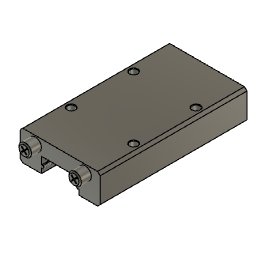
_WozekMGN15H.34389aef-dfec-4a68-be90-59f823977ef3 (Autodesk Fusion 360 design; units mm, degrees)
Autodesk Fusion 360 part; units mm, degrees
sketch "Sketch1" plane through (0, 0, 0) normal (0, 1, 0) x (1, 0, 0)
  line L0 (0, 0) -> (16, 0)
  line L1 (16, 0) -> (16, 12)
  line L2 (16, 12) -> (7.5, 12)
  line L3 (7.5, 6) -> (0, 6)
  line L4 (7.5, 12) -> (7.5, 10)
  line L5 (7.5, 10) -> (7, 10)
  line L6 (6.5, 9.5) -> (6.5, 9.5)
  line L7 (7, 9) -> (7.5, 9)
  line L8 (7.5, 9) -> (7.5, 6)
  arc A0 (6.5, 9.5) -> (7, 9) centre (7, 9.5) ccw
  arc A1 (7, 10) -> (6.5, 9.5) centre (7, 9.5) ccw
  line L9 (-7, 9) -> (-7.5, 9)
  line L10 (-7.5, 10) -> (-7, 10)
  arc A2 (-6.5, 9.5) -> (-7, 10) centre (-7, 9.5) ccw
  arc A3 (-7, 9) -> (-6.5, 9.5) centre (-7, 9.5) ccw
  line L11 (-16, 12) -> (-7.5, 12)
  line L12 (-16, 0) -> (-16, 12)
  line L13 (-6.5, 9.5) -> (-6.5, 9.5)
  line L14 (0, 0) -> (-16, 0)
  line L15 (-7.5, 6) -> (0, 6)
  line L16 (-7.5, 12) -> (-7.5, 10)
  line L17 (-7.5, 9) -> (-7.5, 6)
  point P0 (6.5, 10)
  point P1 (6.5, 9)
  point P2 (-6.5, 9)
  point P3 (-6.5, 10)
  dimension "d1" = 16
  dimension "d2" = 12
  dimension "d3" = 8.5
  dimension "d4" = 6
  dimension "d5" = 7.5
  dimension "d6" = 1
  dimension "d7" = 1
  dimension "d8" = 1
  dimension "d9" = 0.5
  dimension "d10" = 0.5
  constraint coincident L0.start L14.start
  constraint horizontal L0
  constraint perpendicular L0 L1
  constraint perpendicular L1 L2
  constraint perpendicular L2 L4
  constraint perpendicular L4 L5
  constraint perpendicular L3 L8
  constraint coincident P1 L7
  constraint tangent L7 A0
  constraint coincident P0 L5
  constraint coincident P0 L6
  constraint tangent L5 A1
  measures "d1" distance of L0.start L0.end
  measures "d2" distance of L0.end L1.end
  measures "d3" distance of L1.end L2.end
  measures "d4" distance of L2.end L3.start
  measures "d5" distance of L3.start L3.end
  measures "d6" distance of L4.end P0
  measures "d7" distance of P0 P1
  measures "d8" distance of P1 L7.end
  measures "d9" radius of A0
  measures "d10" radius of A1
extrude "Extrude1" add sketch "Sketch1" along normal blind 58.8
sketch "Sketch2" plane through (0, 0, 0) normal (0, 0, 1) x (-1, 0, 0)
  line L0 (16, 0) -> (-16, 0)
  line L1 (-16, 0) -> (-16, -58.8)
  line L2 (-16, -58.8) -> (16, -58.8)
  line L3 (16, -58.8) -> (16, 0)
  line L4 (0, -29.4) -> (-12.5, -29.4)
  line L5 (-12.5, -29.4) -> (-12.5, -41.9)
  line L6 (-12.5, -41.9) -> (0, -41.9)
  line L7 (0, -41.9) -> (0, -29.4)
  circle A0 centre (-12.5, -41.9) radius 1.5
  circle A1 centre (12.5, -41.9) radius 1.5
  circle A2 centre (12.5, -16.9) radius 1.5
  circle A3 centre (-12.5, -16.9) radius 1.5
  dimension "d13" = 12.5
  dimension "d14" = 12.5
  dimension "d15" = 3
  constraint horizontal L4
  constraint vertical L5
  constraint horizontal L6
  constraint vertical L7
  constraint coincident L5.end L6.start
  constraint symmetric L7 A0 A1
  constraint symmetric L4 A0 A3
  constraint symmetric L4 A1 A2
  measures "d13" distance of L4.start L4.end
  measures "d14" distance of L4.start L6.end
  measures "d15" diameter of A0
extrude "Extrude2" cut sketch "Sketch2" against normal blind 6 contours L5 L6 A0 | L5 L6 A0 | A1 | A2 | A3
chamfer "Chamfer1" distance 1 angle 45 4 edges at (-16, 29.4, 0) (-16, 29.4, -12) (16, 29.4, 0) (16, 29.4, -12)
chamfer "Chamfer2" distance 0.2 angle 45 4 edges at (-11.1015, 41.3576, 0) (13.8985, 41.3576, 0) (13.8985, 16.3576, 0) (-11.1015, 16.3576, 0)
sketch "Sketch3" plane through (0, 0, 0) normal (0, -1, 0) x (1, 0, 0)
  line L0 (15, -12) -> (16, -11)
  line L1 (16, -11) -> (16, -1)
  line L2 (16, -1) -> (15, 0)
  line L3 (15, 0) -> (-15, 0)
  line L4 (-15, 0) -> (-16, -1)
  line L5 (-16, -1) -> (-16, -11)
  line L6 (-16, -11) -> (-15, -12)
  line L7 (-15, -12) -> (-7.5, -12)
  line L8 (-7.5, -12) -> (-7.5, -10)
  line L9 (-7.5, -10) -> (-7, -10)
  arc A0 (-7, -10) -> (-7, -9) centre (-7, -9.5) ccw
  line L10 (-7, -9) -> (-7.5, -9)
  line L11 (-7.5, -9) -> (-7.5, -6)
  line L12 (-7.5, -6) -> (7.5, -6)
  line L13 (7.5, -6) -> (7.5, -9)
  line L14 (7.5, -9) -> (7, -9)
  arc A1 (7, -9) -> (7, -10) centre (7, -9.5) ccw
  line L15 (7, -10) -> (7.5, -10)
  line L16 (7.5, -10) -> (7.5, -12)
  line L17 (7.5, -12) -> (15, -12)
  circle A2 centre (-10, -3.0186) radius 2.5
  circle A3 centre (10, -3.0186) radius 2.5
  dimension "d22" = 5
  measures "d22" diameter of A2
extrude "Extrude3" add sketch "Sketch3" along normal blind 4.5 contours A2 | A3
chamfer "Chamfer3" distance 0.5 angle 45 2 edges at (-12.3308, -4.5, -3.9226) (7.6692, -4.5, -3.9226)
sketch "Sketch4" plane through (0, -4.5, 0) normal (0, -1, 0) x (1, 0, 0)
  circle A0 centre (-10, -3.0186) radius 2
  line L0 (-11.0354, -2.0354) -> (-10.9646, -1.9646)
  line L1 (-9.0012, -1.9676) -> (-8.9312, -2.039)
  line L2 (-11.035, -3.9643) -> (-10.965, -4.0357)
  line L3 (-9.0354, -4.0354) -> (-8.9646, -3.9646)
  line L4 (-11.0337, -3.8229) -> (-10.2039, -3.0082)
  line L5 (-9.9898, -2.7981) -> (-9.1426, -1.9663)
  line L6 (-10.8232, -1.9646) -> (-9.9898, -2.7981)
  line L7 (-9.7777, -3.0102) -> (-8.9646, -3.8232)
  line L8 (-10.8236, -4.037) -> (-9.9918, -3.2204)
  line L9 (-9.7777, -3.0102) -> (-8.9325, -2.1804)
  line L10 (-11.0354, -2.1768) -> (-10.2039, -3.0082)
  line L11 (-9.9918, -3.2204) -> (-9.1768, -4.0354)
  arc A1 (-11.0354, -2.0354) -> (-11.0354, -2.1768) centre (-10.9646, -2.1061) ccw
  arc A2 (-10.8232, -1.9646) -> (-10.9646, -1.9646) centre (-10.8939, -2.0354) ccw
  arc A3 (-9.0012, -1.9676) -> (-9.1426, -1.9663) centre (-9.0726, -2.0377) ccw
  arc A4 (-8.9325, -2.1804) -> (-8.9312, -2.039) centre (-9.0025, -2.109) ccw
  arc A5 (-8.9646, -3.9646) -> (-8.9646, -3.8232) centre (-9.0354, -3.8939) ccw
  arc A6 (-9.1768, -4.0354) -> (-9.0354, -4.0354) centre (-9.1061, -3.9646) ccw
  arc A7 (-10.965, -4.0357) -> (-10.8236, -4.037) centre (-10.8936, -3.9656) ccw
  arc A8 (-11.0337, -3.8229) -> (-11.035, -3.9643) centre (-10.9637, -3.8943) ccw
  arc A9 (11.0354, -2.1768) -> (11.0354, -2.0354) centre (10.9646, -2.1061) ccw
  line L12 (11.035, -3.9643) -> (10.965, -4.0357)
  line L13 (9.7777, -3.0102) -> (8.9325, -2.1804)
  line L14 (11.0354, -2.0354) -> (10.9646, -1.9646)
  line L15 (9.9898, -2.7981) -> (9.1426, -1.9663)
  arc A10 (8.9646, -3.8232) -> (8.9646, -3.9646) centre (9.0354, -3.8939) ccw
  arc A11 (8.9312, -2.039) -> (8.9325, -2.1804) centre (9.0025, -2.109) ccw
  line L16 (9.9918, -3.2204) -> (9.1768, -4.0354)
  arc A12 (10.8236, -4.037) -> (10.965, -4.0357) centre (10.8936, -3.9656) ccw
  arc A13 (9.0354, -4.0354) -> (9.1768, -4.0354) centre (9.1061, -3.9646) ccw
  arc A14 (11.035, -3.9643) -> (11.0337, -3.8229) centre (10.9637, -3.8943) ccw
  line L17 (10.8236, -4.037) -> (9.9918, -3.2204)
  arc A15 (9.1426, -1.9663) -> (9.0012, -1.9676) centre (9.0726, -2.0377) ccw
  line L18 (10.8232, -1.9646) -> (9.9898, -2.7981)
  arc A16 (10.9646, -1.9646) -> (10.8232, -1.9646) centre (10.8939, -2.0354) ccw
  line L19 (11.0354, -2.1768) -> (10.2039, -3.0082)
  line L20 (9.0012, -1.9676) -> (8.9312, -2.039)
  line L21 (11.0337, -3.8229) -> (10.2039, -3.0082)
  line L22 (9.7777, -3.0102) -> (8.9646, -3.8232)
  line L23 (9.0354, -4.0354) -> (8.9646, -3.9646)
  point P0 (10, -3.0186)
  dimension "d30" = 0.1
  dimension "d31" = 0.1
  constraint perpendicular L0 L6
  constraint perpendicular L1 L8
  constraint perpendicular L2 L8
  constraint perpendicular L3 L6
  constraint collinear L4 L5
  constraint coincident L7.start L8
  constraint collinear L6 L7
  constraint coincident L8.end L10
  constraint collinear L8 L9
  constraint collinear L10 L11
  constraint tangent L0 A1
  constraint tangent L10 A1
  constraint tangent L0 A2
  constraint tangent L6 A2
  constraint tangent L1 A3
  constraint tangent L5 A3
  constraint equal A2 A3
  constraint tangent L1 A4
  constraint tangent L9 A4
  constraint equal A2 A4
  constraint tangent L3 A5
  constraint tangent L7 A5
  constraint equal A2 A5
  constraint tangent L3 A6
  constraint tangent L11 A6
  constraint equal A2 A6
  constraint tangent L2 A7
  constraint tangent L8 A7
  constraint equal A2 A7
  constraint tangent L2 A8
  constraint tangent L4 A8
  constraint equal A2 A8
  measures "d30" radius of A1
  measures "d31" radius of A2
extrude "Extrude4" cut sketch "Sketch4" against normal blind 1 contours L0 L1 L2 L3 L4 L5 L6 L7 L8 L9 L10 L11 A1 A2 A3 A4 A5 A6 A7 A8 | A9 L12 L13 L14 L15 A10 A11 L16 A12 A13 A14 L17 A15 L18 A16 L19 L20 L21 L22 L23
